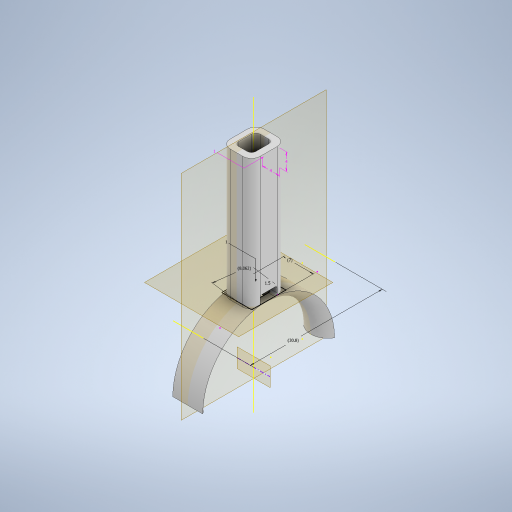
# Autodesk Inventor part: 막대3
Saved by Autodesk Inventor 2023 (Build 270158000, 158)
## iProperties
Created: 2023-04-26
Part Number: 막대3
Material: 일반
Document SubType Name: Modeling
Designer: rlatk
Density: 1 g/cm^3
Appearance: 기본값
Author: rlatk
Autodesk Inventor part; units mm, degrees
ref_plane "XZ Plane" through (0, 0, 0) normal (0, 1, 0) x (-1, 0, 0)
ref_plane "작업 평면1" through (0, 0, 11.4) normal (0, 0, 1) x (1, 0, 0)
sketch "스케치2" plane through (0, 0, 11.4) normal (0, 0, 1) x (1, 0, 0)
  line L0 (-3.8254, 0) -> (3.8254, 0)
  point P0 (0, 0)
  constraints: 2 end point, 1 horizontal
sketch "스케치1" plane through (0, 0, 0) normal (0, 1, 0) x (-1, 0, 0)
  line L0 (0, -4) -> (3.5, -4)
  line L1 (3.5, -4) -> (-3.5, -4)
  arc A0 (3.5, -4) -> (-3.5, -4) centre (0, -5.9365) ccw
  point P0 (0, -1.9365)
  point P1 (-3.5, -4)
  dimension "d0" = 3.5
  dimension "d1" = 3.5
  dimension "d2" = 4
  constraints: 4 end point, 3 point on circle, 1 centre point, 1 midpoint
  measures "d0" distance of L0.start L0.end
  measures "d1" distance of L0.start L1.end
  measures "d2" radius of A0
revolve "회전1" add sketch "스케치1" angle 180 about axis through (-3.8254, 0, 11.4) along (1, 0, 0)
ref_plane "작업 평면2" through (-3.5, 15.4, 11.4) normal (0, 1, 0) x (-1, 0, 0)
sketch "스케치3" plane through (-3.5, 15.4, 11.4) normal (0, 1, 0) x (-1, 0, 0)
  line L0 (0, 15.4) -> (0, -15.4) projected
  line L1 (-7, 11.4) -> (-7, -11.4) projected
  line L2 (0, 4) -> (-7, 4)
  line L3 (-7, 4) -> (-7, -4)
  line L4 (-7, -4) -> (0, -4)
  line L5 (0, -4) -> (0, 4)
  line L6 (-8.8556, 0) -> (1.8556, 0) projected
  point P0 (-3.5, -11.4)
  point P1 (-3.5, 4)
  point P2 (0, -4)
  point P3 (-7, 4)
  dimension "d5" = 4
  dimension "d6" = 4
  constraints: 8 end point, 2 parallel, 2 point on line, 1 horizontal, 1 midpoint, 1 perpendicular
  measures "d5" distance from line of point (-3.5, 4) L6
  measures "d6" distance between parallel lines of L4 L6
extrude "돌출1" add sketch "스케치3" along normal blind 30
sketch "스케치5" plane through (-3.5, 15.4, 11.4) normal (0, 1, 0) x (-1, 0, 0)
  line L0 (-7, -4) -> (0, -4) projected
  line L1 (-7, 4) -> (-7, -4) projected
  line L2 (0, 4) -> (-7, 4) projected
  line L3 (0, -4) -> (0, 4) projected
  line L4 (-7, -4) -> (0, -4)
  line L5 (0, -4) -> (0, 4)
  line L6 (0, 4) -> (-7, 4)
  line L7 (-7, 4) -> (-7, -4)
  line L8 (-2.5, -2.5) -> (-4.5, -2.5)
  line L9 (-5.5, -1.5) -> (-5.5, 1.5)
  line L10 (-4.5, 2.5) -> (-2.5, 2.5)
  line L11 (-1.5, 1.5) -> (-1.5, -1.5)
  arc A0 (-2.5, -2.5) -> (-1.5, -1.5) centre (-2.5, -1.5) ccw
  arc A1 (-1.5, 1.5) -> (-2.5, 2.5) centre (-2.5, 1.5) ccw
  arc A2 (-4.5, 2.5) -> (-5.5, 1.5) centre (-4.5, 1.5) ccw
  arc A3 (-5.5, -1.5) -> (-4.5, -2.5) centre (-4.5, -1.5) ccw
  point P0 (-3.5, -11.4)
  point P1 (-1.5, -2.5)
  point P2 (-5.5, -2.5)
  point P3 (-5.5, 2.5)
  point P4 (-1.5, 2.5)
  dimension "d13" = 1.5
  dimension "d24" = 1
  constraints: 16 end point, 8 point on circle, 8 point on line, 8 tangent, 4 centre point, 3 equal radius, 2 parallel, 1 horizontal, 1 perpendicular, 3 other
  measures "d13" distance between parallel lines of L0 L8
  measures "d24" radius of A0
extrude "돌출3" cut sketch "스케치5" along normal blind 30 and the other way blind 10 contours L8 A3 L9 A2 L10 A1 L11 A0
sketch "스케치6" plane through (3.5, 45.4, 7.4) normal (0, 0, -1) x (-1, 0, 0)
  line L0 (5.5, -31.8494) -> (5.5, -2) projected
  line L1 (2.5, -2) -> (4.5, -2) projected
  line L2 (1.5, -31.8494) -> (1.5, -2) projected
  line L3 (4.5, -2) -> (2.5, -2)
  line L4 (1.5, -3) -> (1.5, -5)
  line L5 (2.5, -6) -> (4.5, -6)
  line L6 (5.5, -5) -> (5.5, -3)
  arc A0 (4.5, -6) -> (5.5, -5) centre (4.5, -5) ccw
  arc A1 (5.5, -3) -> (4.5, -2) centre (4.5, -3) ccw
  arc A2 (2.5, -2) -> (1.5, -3) centre (2.5, -3) ccw
  arc A3 (1.5, -5) -> (2.5, -6) centre (2.5, -5) ccw
  point P0 (3.5, -45.4)
  point P1 (1.5, -6)
  point P2 (1.5, -2)
  point P3 (5.5, -6)
  point P4 (1.5, -6)
  point P5 (5.5, -6)
  point P6 (1.5, -3)
  point P7 (2.5, -2)
  point P8 (5.5, -3)
  point P9 (5.5, -5)
  point P10 (1.5, -5)
  dimension "d18" = 4
  dimension "d19" = 4
  dimension "d23" = 1
  constraints: 8 end point, 8 point on circle, 8 point on line, 8 tangent, 4 centre point, 3 equal radius, 2 parallel, 1 horizontal, 1 perpendicular
  measures "d18" distance of point (5.5, -6) point (1.5, -6)
  measures "d19" distance of point (1.5, -6) point (1.5, -2)
  measures "d23" radius of A0
fillet "모깎기1" radius 2 3 edges at (-3.5, 30.4, 7.4) (3.5, 30.4, 15.4) (-3.5, 30.4, 15.4)
sketch "스케치7" plane through (-3.5, 15.4, 11.4) normal (0, 1, 0) x (-1, 0, 0)
  line L0 (-7, 15.4) -> (0, 15.4) projected
  line L1 (-7, -15.4) -> (0, -15.4) projected
  line L2 (-2, 4) -> (-5, 4) projected
  line L3 (-7, -4) -> (-2, -4) projected
  line L4 (0, -2) -> (0, 2) projected
  line L5 (-7, 2) -> (-7, -4) projected
  point P0 (-3.5, -11.4)
  point P1 (-7, 11.4)
  point P2 (-7, -11.4)
  point P3 (-5, -4)
  point P4 (-3.5, 4)
  point P5 (-4.5, -4)
  point P6 (-7, -2)
  dimension "d27" = 30.8
  dimension "d28" = 8.0623
  dimension "d29" = 7
  constraints: 2 midpoint, 2 other
  measures "d28" distance of point (-3.5, 4) point (-4.5, -4)
  measures "d29" distance between parallel lines of L4 L5
sketch "스케치8" plane through (0, 0, 0) normal (1, 0, 0) x (0, 1, 0)
  line L0 (41.4, 9.4) -> (11.2232, 9.4) projected
  line L1 (15.4, 13.4) -> (45.4, 13.4) projected
  line L2 (11.9081, 9.4) -> (11.9081, 9.4)
  line L3 (12.4081, 9.9) -> (12.4081, 12.9)
  line L4 (11.9081, 13.4) -> (11.9081, 13.4)
  line L5 (11.4081, 12.9) -> (11.4081, 9.9)
  arc A0 (11.9081, 13.4) -> (11.4081, 12.9) centre (11.9081, 12.9) ccw
  arc A1 (12.4081, 12.9) -> (11.9081, 13.4) centre (11.9081, 12.9) ccw
  arc A2 (11.9081, 9.4) -> (12.4081, 9.9) centre (11.9081, 9.9) ccw
  arc A3 (11.4081, 9.9) -> (11.9081, 9.4) centre (11.9081, 9.9) ccw
  point P0 (0, 0)
  point P1 (11.4081, 9.4)
  point P2 (12.4081, 13.4)
  point P3 (11.2232, 13.4)
  point P4 (11.4081, 13.4)
  point P5 (11.4081, 13.4)
  point P6 (12.4081, 9.4)
  dimension "d30" = 1
  dimension "d33" = 0.5
  constraints: 8 end point, 8 point on circle, 8 point on line, 8 tangent, 4 centre point, 3 equal radius, 2 parallel, 1 horizontal, 1 perpendicular
  measures "d30" distance of point (11.408, 13.4) point (12.408, 13.4)
  measures "d33" radius of A0
extrude "돌출6" cut sketch "스케치8" against normal blind 10
sketch "스케치9" plane through (0, 0, 0) normal (1, 0, 0) x (0, 1, 0)
  line L0 (15.3772, 15.4) -> (14.8714, 15.4)
  arc A0 (15.4, 11.4) -> (0, 26.8) centre (0, 11.4) ccw projected
  arc A1 (0, -4) -> (15.4, 11.4) centre (0, 11.4) ccw projected
  line L1 (15.4, 13.4) -> (15.4, 15.4) projected
  line L2 (15.4, 11.4) -> (15.4, 7.4) projected
  line L3 (13.5506, 7.4) -> (43.4, 7.4) projected
  line L4 (45.4, 15.4) -> (15.4, 15.4) projected
  arc A2 (15.4, 11.4) -> (15.3268, 12.9) centre (0, 11.4) ccw projected
  line L5 (15.4, 15.4) -> (15.4, 11.4)
  line L6 (15.4, 11.4) -> (15.4, 7.4)
  arc A3 (15.3268, 9.9) -> (15.4, 11.4) centre (0, 11.4) ccw projected
  line L7 (15.4, 7.4) -> (14.8714, 7.4)
  arc A4 (15.4, 11.4) -> (14.8714, 15.4) centre (0, 11.4) ccw
  arc A5 (14.8714, 7.4) -> (15.4, 11.4) centre (0, 11.4) ccw
  line L8 (14.8714, 15.4) -> (15.4, 15.4)
  line L9 (15.4, 15.4) -> (15.4, 15.4)
  line L10 (15.4, 15.4) -> (15.4, 11.4)
  line L11 (15.4, 11.4) -> (15.4, 7.4)
  line L12 (15.4, 7.4) -> (14.8714, 7.4)
  arc A6 (0, -4) -> (15.4, 11.4) centre (0, 11.4) ccw projected
  arc A7 (14.8714, 7.4) -> (15.4, 11.4) centre (0, 11.4) ccw
  line L13 (14.8714, 7.4) -> (15.4, 7.4)
  line L14 (15.4, 7.4) -> (15.4, 11.4)
  line L15 (15.4, 11.4) -> (15.4, 7.4)
  point P0 (0, 0)
  constraints: 24 end point, 8 point on circle, 6 tangent, 3 centre point, 3 collinear, 3 horizontal, 2 concentric, 2 perpendicular, 1 point on line, 1 vertical
extrude "돌출7" add sketch "스케치9" along normal blind 3.5 and the other way blind 3.5
fillet "모깎기2" radius 2 4 edges at (-3.5, 15.1357, 15.4) (-3.5, 15.1357, 7.4) (3.5, 30.1357, 7.4) (3.5, 15.1357, 15.4)
sketch "스케치10" plane through (0, 0, 0) normal (1, 0, 0) x (0, 1, 0)
  line L0 (0, -4) -> (0, -1.9365) projected
  line L1 (0, 26.8) -> (0, 24.7365) projected
  line L2 (-9.1086, 11.4) -> (54.6517, 11.4) projected
  point P0 (0, 0)
sketch "스케치11" plane through (3.5, 15.2696, 13.4) normal (1, 0, 0) x (0, 0, -1)
  arc A0 (17.4, -15.2696) -> (4, 0) centre (2, -15.2696) ccw projected
  line L0 (3.5, 0) -> (0.5, 0)
  line L1 (0, 0.5) -> (0, 1.5)
  line L2 (0.5, 2) -> (3.5, 2)
  line L3 (4, 1.5) -> (4, 0.5)
  arc A1 (3.5, 0) -> (4, 0.5) centre (3.5, 0.5) ccw
  arc A2 (4, 1.5) -> (3.5, 2) centre (3.5, 1.5) ccw
  arc A3 (0.5, 2) -> (0, 1.5) centre (0.5, 1.5) ccw
  arc A4 (0, 0.5) -> (0.5, 0) centre (0.5, 0.5) ccw
  point P0 (13.4, -15.2696)
  point P1 (0, 2)
  point P2 (0, 0)
  point P3 (4, 2)
  dimension "d44" = 4
  dimension "d45" = 2
  dimension "d46" = 0.5
  constraints: 8 end point, 8 point on circle, 8 point on line, 8 tangent, 4 centre point, 3 equal radius, 2 parallel, 1 horizontal, 1 perpendicular
  measures "d44" distance of point (0, 2) point (4, 2)
  measures "d45" distance of point (0, 0) point (0, 2)
  measures "d46" radius of A1
extrude "돌출8" cut sketch "스케치11" against normal blind 3.5
extrude "돌출9" add sketch "스케치5" along normal blind 3.5 contours L8 A3 L9 A2 L10 A1 L11 A0
extrude "돌출10" cut sketch "스케치5" along normal blind 30 contours L8 A3 L9 A2 L10 A1 L11 A0
extrude "돌출11" cut sketch "스케치5" along normal blind 30 and the other way blind 5 contours L8 A3 L9 A2 L10 A1 L11 A0
